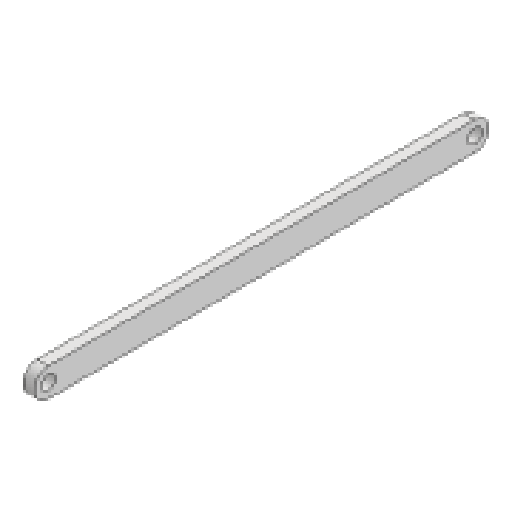
# Autodesk Inventor part: CarrigeSideLinkage
Saved by Autodesk Inventor 2023 (Build 270158000, 158)
## iProperties
Created: 2022-11-08
Part Number: CarrigeSideLinkage
Material: Generic
Document SubType Name: Modeling
Designer: deli
Density: 1 g/cm^3
Appearance: Default
Author: deli
Autodesk Inventor part; units mm, degrees
ref_plane "YZ Plane" through (0, 0, 0) normal (1, 0, 0) x (0, 1, 0)
ref_plane "XZ Plane" through (0, 0, 0) normal (0, 1, 0) x (-1, 0, 0)
ref_plane "XY Plane" through (0, 0, 0) normal (0, 0, 1) x (1, 0, 0)
sketch "Sketch1" plane through (0, 0, 0) normal (1, 0, 0) x (0, 1, 0)
  circle A0 centre (-152.2127, -77.2775) radius 2
  arc A1 (-148.2132, -77.3388) -> (-156.2127, -77.2775) centre (-152.2127, -77.2775) ccw
  line L0 (-148.2132, -77.2162) -> (-148.2132, -218.7162)
  circle A2 centre (-152.2132, -218.7162) radius 2
  arc A3 (-156.2132, -218.7162) -> (-148.2132, -218.7162) centre (-152.2132, -218.7162) ccw
  line L1 (-156.2127, -77.2775) -> (-156.2132, -218.7162)
  point P0 (0, 0)
  dimension "d0" = 4
  dimension "d1" = 8
  dimension "d2" = 141.5
  constraints: 5 point on circle, 4 centre point, 4 end point, 3 tangent, 2 coincident, 2 equal radius, 1 point on line, 1 vertical
  measures "d0" diameter of A0
  measures "d1" diameter of A1
  measures "d2" distance of L0.start L0.end
extrude "Extrusion1" add sketch "Sketch1" along normal blind 3.175
body "Solid1"
